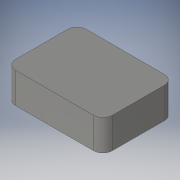
# Autodesk Inventor part: Case
Saved by Autodesk Inventor 2016 (Build 200138000, 138)
## iProperties
Created: 2016-03-25
Part Number: Case
Material: PC/ABS Plastic
Document SubType Name: Modeling
Designer: agmle
Density: 0.357273 g/cm^3
Appearance: Smooth - Medium Gray
Mass: 1360.01 g
Surface Area: 5129.52 cm^2
Volume: 3806.64 cm^3
Inside_Height: 10.238 in
Inside_Depth: 4.366 in
Draft_Angle: 1.50 deg
Horizontal_Inside_Radius: 0.388 in
Boss_Draft_Z: 0.320 in
Author: agmle
Autodesk Inventor part; units mm, degrees
ref_plane "YZ Plane" through (0, 0, 0) normal (1, 0, 0) x (0, 1, 0)
ref_plane "XZ Plane" through (0, 0, 0) normal (0, 1, 0) x (-1, 0, 0)
ref_plane "XY Plane" through (0, 0, 0) normal (0, 0, 1) x (1, 0, 0)
sketch "Sketch1" plane through (0, 0, 0) normal (0, 1, 0) x (-1, 0, 0)
  line L0 (182.88, -49.7078) -> (180.0606, -49.7078)
  line L1 (180.0606, -49.7078) -> (180.0606, 49.7078)
  line L2 (180.0606, 49.7078) -> (182.88, 49.7078)
  line L3 (-180.0606, -49.7078) -> (-182.88, -49.7078)
  line L4 (-182.88, 49.7078) -> (-180.0606, 49.7078)
  line L5 (-180.0606, 49.7078) -> (-180.0606, -49.7078)
  line L6 (-102.9589, -130.0226) -> (-102.9589, -127.2032)
  line L7 (-102.9589, -127.2032) -> (102.9589, -127.2032)
  line L8 (102.9589, -127.2032) -> (102.9589, -130.0226)
  line L9 (18.4277, 130.0226) -> (18.4277, 127.2032)
  line L10 (18.4277, 127.2032) -> (102.9589, 127.2032)
  line L11 (102.9589, 127.2032) -> (102.9589, 130.0226)
  line L12 (-18.4277, 127.2032) -> (-102.9589, 127.2032)
  line L13 (-102.9589, 127.2032) -> (-102.9589, 130.0226)
  line L14 (-18.4277, 130.0226) -> (-18.4277, 127.2032)
  line L15 (18.4277, 128.6129) -> (-18.4277, 128.6129) construction
  line L16 (182.88, -130.0226) -> (102.9589, -130.0226)
  line L17 (-102.9589, -130.0226) -> (-182.88, -130.0226)
  line L18 (102.9589, 130.0226) -> (182.88, 130.0226)
  line L19 (-182.88, -130.0226) -> (-182.88, -49.7078)
  line L20 (-182.88, 49.7078) -> (-182.88, 130.0226)
  line L21 (182.88, 130.0226) -> (182.88, 49.7078)
  line L22 (182.88, -49.7078) -> (182.88, -130.0226)
  line L23 (-182.88, 130.0226) -> (-102.9589, 130.0226)
  line L24 (-18.4277, 130.0226) -> (18.4277, 130.0226)
  line L25 (182.88, -130.0226) -> (-182.88, 130.0226) construction
  line L26 (-182.88, -130.0226) -> (182.88, 130.0226) construction
  line L27 (196.85, -143.9926) -> (-196.85, -143.9926)
  line L28 (-196.85, -143.9926) -> (-196.85, 143.9926)
  line L29 (-196.85, 143.9926) -> (196.85, 143.9926)
  line L30 (196.85, 143.9926) -> (196.85, -143.9926)
  line L31 (182.88, -89.8652) -> (196.85, -89.8652) construction
  line L32 (182.88, 89.8652) -> (196.85, 89.8652) construction
  line L33 (-182.88, 89.8652) -> (-196.85, 89.8652) construction
  line L34 (-182.88, -89.8652) -> (-196.85, -89.8652) construction
  line L35 (-142.9195, -130.0226) -> (-142.9195, -143.9926) construction
  line L36 (142.9195, -130.0226) -> (142.9194, -143.9926) construction
  line L37 (142.9195, 130.0226) -> (142.9194, 143.9926) construction
  line L38 (-142.9195, 130.0226) -> (-142.9195, 143.9926) construction
  point P0 (0, 0)
  point P1 (180.0606, 0)
  point P2 (0, 128.6129)
  point P3 (0, -127.2032)
  point P4 (0, 0)
  dimension "Inside_Height" = 260.0452
  dimension "Inside_Width" = 365.76
  dimension "Boss_Draft_X" = 2.8194
  dimension "Side_Boss_Width" = 99.4156
  dimension "Front_Boss_Width" = 84.5312
  dimension "Front_Boss_Gap" = 36.8554
  dimension "Wall_Thickness" = 13.97
  constraints: 78 end point, 18 parallel, 17 point on line, 15 equal length, 14 midpoint, 11 perpendicular, 6 horizontal, 3 collinear, 1 coincident
  measures "Inside_Height" distance of L18.end L16.start
  measures "Inside_Width" distance of L16.start L17.end
  measures "Boss_Draft_X" distance of L6.start L6.end
  measures "Side_Boss_Width" distance of L0.end L1.end
  measures "Front_Boss_Width" distance of L9.end L10.end
  measures "Front_Boss_Gap" distance of L15.start L15.end
  measures "Wall_Thickness" distance of L31.start L31.end
extrude "Extrusion1" add sketch "Sketch1" along normal blind 110.8964
sketch "Sketch2" plane through (0, 110.8964, 0) normal (0, 1, 0) x (1, 0, 0)
  line L0 (-196.85, -143.9926) -> (196.85, -143.9926) projected
  line L1 (-196.85, 143.9926) -> (-196.85, -143.9926) projected
  line L2 (196.85, 143.9926) -> (-196.85, 143.9926) projected
  line L3 (196.85, -143.9926) -> (196.85, 143.9926) projected
  point P0 (0, 0)
extrude "Extrusion2" add sketch "Sketch2" along normal blind 13.97
chamfer "Chamfer1" distance 2.8194 distance2 8.128 1 edges at (60.6933, 0, 127.2032) measured on face at (60.6933, 0, 127.7032)
chamfer "Chamfer2" distance 2.8194 distance2 8.128 1 edges at (-60.6933, 0, 127.2032) measured on face at (-60.6933, 0, 127.7032)
chamfer "Chamfer3" distance 2.8194 distance2 8.128 1 edges at (-180.0606, 0, 0) measured on face at (-180.5606, 0, 0)
chamfer "Chamfer4" distance 2.8194 distance2 8.128 1 edges at (0, 0, -127.2032) measured on face at (0, 0, -127.7032)
chamfer "Chamfer5" distance 2.8194 distance2 8.128 1 edges at (180.0606, 0, 0) measured on face at (180.5606, 0, 0)
fillet "Fillet1" radius 24.13 4 edges at (-182.88, 55.4482, -130.0226) (182.88, 55.4482, -130.0226) (182.88, 55.4482, 130.0226) (-182.88, 55.4482, 130.0226)
fillet "Fillet2" radius 38.1 4 edges at (-196.85, 62.4332, -143.9926) (196.85, 62.4332, -143.9926) (196.85, 62.4332, 143.9926) (-196.85, 62.4332, 143.9926)
draft "FaceDraft1" angle 1.5 pull direction (0, -1, 0) fixed plane through (34.3196, 0, -139.3359) normal (0, -1, 0) faces at (121.5559, 36.9655, -130.0226) (170.815, 36.9655, -126.7898) (182.88, 73.9309, -68.4361) (182.88, 36.9655, 68.4361) (160.5532, 36.9655, 129.9551) (140.153, 36.9655, 130.0226) (-6.1426, 73.9309, 130.0226) (-121.5559, 36.9655, 130.0226) (-172.3429, 36.9655, 125.8297) (-182.88, 73.9309, 87.1643) (-140.153, 36.9655, -130.0226) (-167.5657, 36.9655, -128.3546) (-182.88, 73.9309, -68.4361)
fillet "Fillet3" radius 9.8552 18 edges at (-173.7591, 110.8964, 120.9017) (-179.9761, 110.8964, -77.8002) (-179.9761, 110.8964, 0) (-179.9761, 110.8964, 77.8002) (-173.7591, 110.8964, -120.9017) (130.8544, 110.8964, -127.1187) (-130.8545, 110.8964, -127.1187) (0, 110.8964, -127.1187) (173.7591, 110.8964, -120.9017) (179.9761, 110.8964, -77.8002) (179.9761, 110.8964, 0) (179.9761, 110.8964, 77.8002) (173.7591, 110.8964, 120.9017) (130.8545, 110.8964, 127.1187) (-130.8544, 110.8964, 127.1187) (60.6933, 110.8964, 127.1187) (0, 110.8964, 127.1187) (-60.6933, 110.8964, 127.1187)
sketch "Sketch3" plane through (0, 110.8964, 0) normal (0, -1, 0) x (1, 0, 0)
  line L0 (103.4098, -63.5) -> (-103.4098, -63.5)
  line L1 (-115.0938, -51.816) -> (-115.0938, 51.816)
  line L2 (-103.4098, 63.5) -> (103.4098, 63.5)
  line L3 (115.0937, 51.816) -> (115.0937, -51.816)
  line L4 (0, -63.5) -> (0, 63.5) construction
  line L5 (103.4098, -63.5) -> (115.0937, -51.816)
  line L6 (-103.4098, -63.5) -> (-115.0938, -51.816)
  line L7 (-115.0938, 51.816) -> (-103.4098, 63.5)
  line L8 (103.4098, 63.5) -> (115.0937, 51.816)
  point P0 (0, 0)
  point P1 (0, 0)
  dimension "d36" = 230.1875
  dimension "d37" = 127
  dimension "d38" = 11.684
  dimension "d39" = 11.684
  constraints: 18 end point, 6 perpendicular, 5 midpoint, 3 parallel, 2 point on line, 1 coincident, 1 horizontal
  measures "d36" distance between parallel lines of L1 L3
  measures "d37" distance between parallel lines of L2 L0
  measures "d38" distance from line of L0.start L3
  measures "d39" distance from line of L3.end L0
extrude "Extrusion3" add sketch "Sketch3" along normal blind 2.032
equation "\"d11\" = Wall_Thickness"
equation "\"d13\" = Boss_Draft_X"
equation "\"d16\" = Boss_Draft_X"
equation "\"d17\" = Boss_Draft_Z"
equation "\"d19\" = Boss_Draft_X"
equation "\"d20\" = Boss_Draft_Z"
equation "\"d22\" = Boss_Draft_X"
equation "\"d23\" = Boss_Draft_Z"
equation "\"d25\" = Boss_Draft_X"
equation "\"d26\" = Boss_Draft_Z"
equation "\"Boss_Draft_Z\" = 8.128"
body "Solid1"
